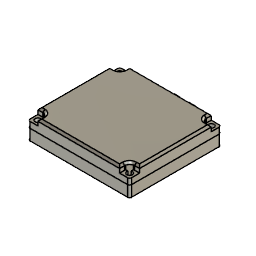
tgam_holder v1 (Autodesk Fusion 360 design; units mm, degrees)
Autodesk Fusion 360 part; units mm, degrees
note: some values were not read from the file. Set by a fixed rule: which sketch regions a step uses.
sketch "Sketch1" plane through (0, 0, 0) normal (0, 0, 1) x (1, 0, 0)
  line L0 (-40, 40) -> (5, 40)
  line L1 (5, 40) -> (5, 0)
  line L2 (5, 0) -> (-40, 0)
  line L3 (-40, 0) -> (-40, 40)
  dimension "d1" = 45
  dimension "d2" = 40
  constraint horizontal L0
  constraint vertical L1
  constraint horizontal L2
  constraint vertical L3
  measures "d1" distance of L0.start L0.end
  measures "d2" distance of L0.start L2.end
extrude "Extrude1" add sketch "Sketch1" along normal blind 10 makes body 1
sketch "Sketch2" plane through (0, 0, 10) normal (0, 0, 1) x (-1, 0, 0)
  line L0 (40, 0) -> (-5, 0)
  line L1 (-5, 0) -> (-5, -40)
  line L2 (-5, -40) -> (40, -40)
  line L3 (40, -40) -> (40, 0)
  line L4 (43, 3) -> (-8, 3)
  line L5 (-8, 3) -> (-8, -43)
  line L6 (-8, -43) -> (43, -43)
  line L7 (43, -43) -> (43, 3)
  dimension "d5" = 3
extrude "Extrude2" add sketch "Sketch2" against normal blind 10 separate body makes body 2
extrude "Extrude3" add 2 faces at (-10, -2, 10) (-25, 13.3333, 10) along direction (0, 0, 1) blind 3 on bodies 1 2 bodies 2
sketch "Sketch3" plane through (0, 0, 0) normal (0, 0, -1) x (1, 0, 0)
  line L0 (-40, -40) -> (-40, 0)
  line L1 (-40, 0) -> (5, 0)
  line L2 (5, 0) -> (5, -40)
  line L3 (5, -40) -> (-40, -40)
  line L4 (-43, 3) -> (-43, -43)
  line L5 (-43, -43) -> (8, -43)
  line L6 (8, -43) -> (8, 3)
  line L7 (8, 3) -> (-43, 3)
  line L8 (5, -40) -> (-40, -40)
  line L9 (-40, -40) -> (-40, 0)
  line L10 (-40, 0) -> (5, 0)
  line L11 (5, 0) -> (5, -40)
  dimension "d10" = 0
  measures "d10" distance of L1
extrude "Extrude4" add sketch "Sketch3" along normal blind 3 contours L0 L1 L2 L3 L8 L9 L10 L11 | L4 L5 L6 L7 bodies 2
sketch "Sketch4" plane through (0, 0, 13) normal (0, 0, 1) x (-1, 0, 0)
  line L0 (43, -43) -> (43, 3)
  line L1 (43, 3) -> (-8, 3)
  line L2 (-8, 3) -> (-8, -43)
  line L3 (-8, -43) -> (43, -43)
  line L4 (19, -43) -> (19, 3)
  line L5 (-8, -37) -> (19, -37)
  line L6 (19, -3) -> (-8, -3)
  line L7 (-2, -37) -> (-2, -3)
  dimension "d13" = 27
  dimension "d14" = 6
  dimension "d15" = 6
  dimension "d16" = 6
  constraint coincident L3 L4.start
  constraint perpendicular L3 L4
  constraint coincident L1 L4.end
  constraint coincident L2 L5.start
  constraint coincident L4 L5.end
  constraint perpendicular L4 L5
  constraint coincident L4 L6.start
  constraint coincident L2 L6.end
  constraint perpendicular L2 L6
  constraint coincident L5 L7.start
  constraint coincident L6 L7.end
  constraint perpendicular L6 L7
  measures "d13" distance of L2 L4
  measures "d14" distance of L3 L5
  measures "d15" distance of L1 L6
  measures "d16" distance of L2 L7
extrude "Extrude5" cut sketch "Sketch4" against normal blind 3 contours L4 L5 L6 L7 bodies 2
ref_plane "WorkPlane1" through (-17.5, 20, 5) normal (0, 0, 1) x (1, 0, 0)
split "Split1" by plane through (-17.5, 20, 5) normal (0, 0, 1) bodies 2 makes body 3 at (-35, 25.6667, 13)
sketch "Sketch5" plane through (-43, 0, 0) normal (-1, 0, 0) x (0, -1, 0)
  line L0 (3, 5) -> (-43, 5)
  line L1 (-43, 5) -> (-43, -3)
  line L2 (-43, -3) -> (3, -3)
  line L3 (3, -3) -> (3, 5)
  line L4 (-43, -3) -> (-49.2, -3)
  line L5 (-51, -1.2) -> (-51, 0.2)
  line L6 (-49.2, 2) -> (-43, 2)
  line L7 (-43, 2) -> (-43, -3)
  line L8 (-43, -0.5) -> (-51, -0.5)
  circle A0 centre (-49, -0.5) radius 1.4
  line L9 (-51, -1.2) -> (-49.2, -3)
  line L10 (-49.2, 2) -> (-51, 0.2)
  point P0 (-51, -3)
  point P1 (-51, 2)
  point P2 (-43, -0.5)
  dimension "d20" = 8
  dimension "d21" = 5
  dimension "d22" = 2.8
  dimension "d23" = 1.8
  dimension "d24" = 1.8
  dimension "d25" = 1.8
  dimension "d26" = 1.8
  constraint horizontal L4
  constraint vertical L5
  constraint horizontal L6
  constraint vertical L7
  constraint coincident L1.end L2.start
  constraint midpoint L7 P2
  constraint coincident P2 L8.start
  constraint coincident L8 A0.centre
  constraint coincident L5 L8.end
  constraint coincident P0 L5
  constraint coincident P0 L4
  constraint coincident P1 L6
  constraint coincident P1 L5
  measures "d20" distance of L1.end P0
  measures "d21" distance of L1.end L6.end
  measures "d22" diameter of A0
  measures "d23" distance of P0 L5.start
  measures "d24" distance of P0 L4.end
  measures "d25" distance of P1 L6.start
  measures "d26" distance of P1 L5.end
extrude "Extrude6" add 1 faces at (2, 25.6667, 11) along direction (-1, 0, 0) blind 25 on bodies 3 bodies 3
sketch "Sketch6" plane through (-43, 0, 0) normal (-1, 0, 0) x (0, -1, 0)
  line L0 (-43, 5) -> (3, 5)
  line L1 (3, 5) -> (3, 13)
  line L2 (3, 13) -> (-43, 13)
  line L3 (-43, 13) -> (-43, 5)
  line L4 (-40, 13) -> (-40, -3)
  line L5 (-43, 2) -> (-43, -3)
  line L6 (-43, 10) -> (3, 10)
  line L7 (3, 0) -> (-43, 0)
  line L8 (-43, -3) -> (3, -3)
  line L9 (-35, 8) -> (-22, 8)
  line L10 (-22, 8) -> (-22, 2)
  line L11 (-22, 2) -> (-35, 2)
  line L12 (-35, 2) -> (-35, 8)
  dimension "d29" = 3
  dimension "d30" = 3
  dimension "d31" = 3
  constraint coincident L2 L4.start
  constraint perpendicular L0 L4
  constraint coincident L3 L6.start
  constraint coincident L1 L6.end
  constraint perpendicular L1 L6
  constraint coincident L5 L7.end
  constraint perpendicular L5 L7
  constraint horizontal L9
  constraint vertical L10
  constraint horizontal L11
  constraint vertical L12
  measures "d29" distance of L4 L5
  measures "d30" distance of L2 L6
  measures "d31" distance of L7 L8
extrude "Extrude7" cut sketch "Sketch6" against normal blind 3 contours L0 L9 L10 L12 | L0 L10 L11 L12 bodies 2 3
sketch "Sketch7" plane through (0, 43, 0) normal (0, 1, 0) x (-1, 0, 0)
  line L0 (-8, 5) -> (43, 5)
  line L1 (43, 5) -> (43, 13)
  line L2 (43, 13) -> (-8, 13)
  line L3 (-8, 13) -> (-8, 5)
  line L4 (14.5, 13) -> (14.5, -3)
  line L5 (20.5, 13) -> (20.5, -3)
  line L6 (17.5, 13) -> (17.5, -3)
  line L7 (13, 5) -> (13, -3)
  line L8 (22, 5) -> (22, -3)
  point P0 (17.5, 13)
  dimension "d34" = 3
  dimension "d35" = 3
  dimension "d36" = 1.5
  dimension "d37" = 1.5
  constraint midpoint L2 P0
  constraint coincident L2 L4.start
  constraint perpendicular L0 L4
  constraint coincident L2 L5.start
  constraint perpendicular L2 L5
  constraint coincident P0 L6.start
  constraint perpendicular L0 L6
  constraint coincident L0 L7.start
  constraint perpendicular L0 L7
  constraint coincident L0 L8.start
  constraint perpendicular L0 L8
  measures "d34" distance of L4 L6
  measures "d35" distance of L5 L6
  measures "d36" distance of L4 L7
  measures "d37" distance of L5 L8
extrude "Extrude8" add sketch "Sketch5" against normal blind 1.5 from surface at -21 contours L1 L5 L6 L7 L8 A0 L10 | L1 L4 L5 L7 L8 A0 L9 bodies 2
extrude "Extrude9" add sketch "Sketch5" against normal blind 1.5 from surface at -28.5 contours L1 L5 L6 L7 L8 A0 L10 | L1 L4 L5 L7 L8 A0 L9 bodies 2
sketch "Sketch8" plane through (0, 0, 13) normal (0, 0, 1) x (-1, 0, 0)
  line L0 (43, -43) -> (43, 3)
  line L1 (43, 3) -> (-8, 3)
  line L2 (-8, 3) -> (-8, -43)
  line L3 (-8, -43) -> (43, -43)
  circle A0 centre (-5.5, 0.5) radius 1.4
  circle A1 centre (40.5, 0.5) radius 1.4
  line L4 (-8, -20) -> (43, -20)
  circle A2 centre (-5.5, -40.5) radius 1.4
  circle A3 centre (40.5, -40.5) radius 1.4
  line L5 (-3, -40.5) -> (-3, -43)
  line L6 (40.5, -2) -> (43, -2)
  line L7 (38, 3) -> (38, 0.5)
  line L8 (-8, -38) -> (-5.5, -38)
  arc A4 (-3, -40.5) -> (-5.5, -38) centre (-5.5, -40.5) ccw
  arc A5 (38, 0.5) -> (40.5, -2) centre (40.5, 0.5) ccw
  line L9 (-8, -2) -> (-5.5, -2)
  arc A6 (-5.5, -2) -> (-3, 0.5) centre (-5.5, 0.5) ccw
  line L10 (-3, 0.5) -> (-3, 3)
  arc A7 (40.5, -38) -> (38, -40.5) centre (40.5, -40.5) ccw
  line L11 (38, -43) -> (38, -40.5)
  line L12 (40.5, -38) -> (43, -38)
  dimension "d44" = 2.8
  dimension "d45" = 2.8
  dimension "d46" = 2.5
  dimension "d47" = 2.5
  dimension "d48" = 2.5
  dimension "d49" = 2.5
  dimension "d52" = 5
  dimension "d53" = 5
  dimension "d54" = 5
  dimension "d55" = 5
  dimension "d68" = 2.5
  dimension "d69" = 2.5
  constraint midpoint L2 L4.start
  constraint midpoint L0 L4.end
  constraint symmetric A0 L4 A2
  constraint symmetric A1 L4 A3
  constraint coincident L3 L5.end
  constraint perpendicular L3 L5
  constraint coincident L0 L6.end
  constraint perpendicular L0 L6
  constraint coincident L1 L7.start
  constraint perpendicular L3 L7
  constraint coincident L2 L8.start
  constraint perpendicular L0 L8
  constraint tangent L5 A4
  constraint tangent L8 A4
  constraint tangent L6 A5
  constraint tangent L7 A5
  constraint symmetric L4 L5.end L10.end
  constraint symmetric L4 L6.end L12.end
  constraint symmetric L4 L7.start L11.start
  constraint symmetric L4 L8.start L9.start
  constraint symmetric L4 L5.start A6.end
  constraint symmetric L4 L8.end L9.end
  constraint symmetric L4 A4 A6
  constraint symmetric L4 L6.start A7.start
  constraint symmetric L4 L7.end A7.end
  constraint symmetric L4 A5 A7
  measures "d44" diameter of A0
  measures "d45" diameter of A1
  measures "d46" distance of L1 A0.centre
  measures "d47" distance of L2 A0.centre
  measures "d48" distance of L1 A1.centre
  measures "d49" distance of L0 A1.centre
  measures "d52" distance of L2 L5
  measures "d53" distance of L1 L6
  measures "d54" distance of L0 L7
  measures "d55" distance of L3 L8
  measures "d68" radius of A4
  measures "d69" radius of A5
extrude "Extrude10" cut sketch "Sketch8" against normal blind 19 contours A0 | A1 | A2 | A3 bodies 2 3
extrude "Extrude11" cut sketch "Sketch5" against normal blind 100 contours L1 L5 L6 L7 L8 A0 L10 | L1 L4 L5 L7 L8 A0 L9 bodies 2
extrude "Extrude12" add sketch "Sketch5" against normal blind 1.5 from surface at -21 separate body contours L1 L5 L6 L7 L8 A0 L10 | L1 L4 L5 L7 L8 A0 L9 makes body 4
extrude "Extrude13" add sketch "Sketch5" against normal blind 1.5 from surface at -28.5 separate body contours L1 L5 L6 L7 L8 A0 L10 | L1 L4 L5 L7 L8 A0 L9 makes body 5
move_body "Move1" bodies 5 4 to x (1, 0, 0) y (0, 1, 0) z (0, 0, 1) at (0, 0, 2)
extrude "Extrude14" cut 1 faces at (-24.8246, 13.4841, -3) along direction (0, 0, 1) blind 2 on bodies 2 bodies 2
extrude "Extrude15" cut sketch "Sketch8" against normal blind 2 bodies 3
extrude "Extrude16" cut sketch "Sketch8" against normal blind 5 contours L0 L3 A7 L11 L12 | L2 L3 L5 L8 A4 | L0 L1 L6 L7 A5 | L1 L2 L9 A6 L10 bodies 3
fillet "Fillet1" radius 1 8 edges at (8, -3, 2) (8, 43, 2) (-43, 43, 2) (-43, -3, 2) (8, -3, 6.5) (8, 43, 6.5) (-43, 43, 6.5) (-43, -3, 6.5) on bodies 2 3
chamfer "Chamfer1" distance 1 angle 45 16 edges at (-17.5, -3, 11) (-38.7322, 1.2678, 11) (-38, -1.75, 11) (-41.75, 2, 11) (-43, 20, 11) (-38.7322, 38.7322, 11) (-41.75, 38, 11) (-38, 41.75, 11) (-17.5, 43, 11) (3.7322, 38.7322, 11) (3, 41.75, 11) (6.75, 38, 11) (8, 20, 11) (3.7322, 1.2678, 11) (6.75, 2, 11) (3, -1.75, 11) on bodies 3
combine "Combine1" operation add target body 2 tool bodies 5 4
fillet "Fillet2" radius 0.5 14 edges at (-32, 43, -1) (-42.7071, 42.7071, -1) (-43, 20, -1) (-42.7071, -2.7071, -1) (-17.5, -3, -1) (7.7071, -2.7071, -1) (8, 20, -1) (7.7071, 42.7071, -1) (-3, 43, -1) (-13, 46.1, -1) (-14.5, 46.1, -1) (-20.5, 46.1, -1) (-22, 46.1, -1) (-17.5, 43, -1) on bodies 2
sketch "Sketch9" plane through (0, 43, 0) normal (0, 1, 0) x (-1, 0, 0)
  line L0 (38, 10) -> (-3, 10)
  line L1 (-3, 10) -> (-3, 8)
  line L2 (-3, 8) -> (-7, 8)
  line L3 (-7, 8) -> (-7, 5)
  line L4 (-7, 5) -> (42, 5)
  line L5 (42, 5) -> (42, 8)
  line L6 (42, 8) -> (38, 8)
  line L7 (38, 8) -> (38, 10)
  circle A0 centre (6, 5) radius 3.5
  dimension "d77" = 7
  constraint coincident L4 A0.centre
  measures "d77" diameter of A0
extrude "Extrude17" cut sketch "Sketch9" against normal blind 3 contours L4 A0 | L4 A0 bodies 2 3
copy_body "Body->Comp1" bodies 2 removing the originals makes body 6 in component "Component"
copy_body "Body->Comp2" bodies 3 removing the originals makes body 7 in component "Component'"
component "Component" placed x (1, 0, 0) y (0, 1, 0) z (0, 0, 1) at (0, 0, 0)
component "Component'" placed x (1, 0, 0) y (0, 1, 0) z (0, 0, 1) at (0, 0, 0)
hidden bodies 1
equation "d24 = d23"
equation "d26 = d25"
